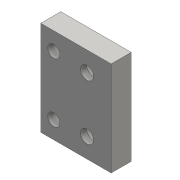
# Autodesk Inventor part: ROB-R-J-1
Saved by Autodesk Inventor 2016 (Build 200138000, 138)
## iProperties
Created: 2016-02-12
Part Number: ROB-R-J-1
Material: Generic
Document SubType Name: Modeling
Designer: admin
Density: 1 g/cm^3
Appearance: Default
Author: admin
Autodesk Inventor part; units mm, degrees
(part 1 of 3)
ref_plane "YZ Plane" through (0, 0, 0) normal (1, 0, 0) x (0, 1, 0)
ref_plane "XZ Plane" through (0, 0, 0) normal (0, 1, 0) x (-1, 0, 0)
ref_plane "XY Plane" through (0, 0, 0) normal (0, 0, 1) x (1, 0, 0)
sketch "Sketch1" plane through (0, 0, 0) normal (0, 1, 0) x (-1, 0, 0)
  spline S0 degree 3 poles (-66.561, 0) (-66.561, -4.1087) (-69.8644, -7.4121) (-73.9731, -7.4121) knots 0 0 0 0 1 1 1 1
  line L0 (-66.561, 0) -> (-66.561, -4.1087) construction
  line L1 (-66.561, -4.1087) -> (-69.8644, -7.4121) construction
  line L2 (-69.8644, -7.4121) -> (-73.9731, -7.4121) construction
  spline S1 degree 3 poles (-73.9731, -7.4121) (-78.0818, -7.4121) (-81.3852, -4.1087) (-81.3852, 0) knots 0 0 0 0 1 1 1 1
  line L3 (-73.9731, -7.4121) -> (-78.0818, -7.4121) construction
  line L4 (-78.0818, -7.4121) -> (-81.3852, -4.1087) construction
  line L5 (-81.3852, -4.1087) -> (-81.3852, 0) construction
  spline S2 degree 3 poles (-81.3852, 0) (-81.3852, 4.1087) (-78.0818, 7.4121) (-73.9731, 7.4121) knots 0 0 0 0 1 1 1 1
  line L6 (-81.3852, 0) -> (-81.3852, 4.1087) construction
  line L7 (-81.3852, 4.1087) -> (-78.0818, 7.4121) construction
  line L8 (-78.0818, 7.4121) -> (-73.9731, 7.4121) construction
  spline S3 degree 3 poles (-73.9731, 7.4121) (-69.8644, 7.4121) (-66.561, 4.1087) (-66.561, 0) knots 0 0 0 0 1 1 1 1
  line L9 (-73.9731, 7.4121) -> (-69.8644, 7.4121) construction
  line L10 (-69.8644, 7.4121) -> (-66.561, 4.1087) construction
  line L11 (-66.561, 4.1087) -> (-66.561, 0) construction
  spline S4 degree 3 poles (74.4391, 0) (74.4391, -4.1087) (71.1356, -7.4121) (67.027, -7.4121) knots 0 0 0 0 1 1 1 1
  line L12 (74.4391, 0) -> (74.4391, -4.1087) construction
  line L13 (74.4391, -4.1087) -> (71.1356, -7.4121) construction
  line L14 (71.1356, -7.4121) -> (67.027, -7.4121) construction
  spline S5 degree 3 poles (67.027, -7.4121) (62.9183, -7.4121) (59.6149, -4.1087) (59.6149, 0) knots 0 0 0 0 1 1 1 1
  line L15 (67.027, -7.4121) -> (62.9183, -7.4121) construction
  line L16 (62.9183, -7.4121) -> (59.6149, -4.1087) construction
  line L17 (59.6149, -4.1087) -> (59.6149, 0) construction
  spline S6 degree 3 poles (59.6149, 0) (59.6149, 4.1087) (62.9183, 7.4121) (67.027, 7.4121) knots 0 0 0 0 1 1 1 1
  line L18 (59.6149, 0) -> (59.6149, 4.1087) construction
  line L19 (59.6149, 4.1087) -> (62.9183, 7.4121) construction
  line L20 (62.9183, 7.4121) -> (67.027, 7.4121) construction
  spline S7 degree 3 poles (67.027, 7.4121) (71.1356, 7.4121) (74.4391, 4.1087) (74.4391, 0) knots 0 0 0 0 1 1 1 1
  line L21 (67.027, 7.4121) -> (71.1356, 7.4121) construction
  line L22 (71.1356, 7.4121) -> (74.4391, 4.1087) construction
  line L23 (74.4391, 4.1087) -> (74.4391, 0) construction
  spline S8 degree 3 poles (-60.9702, 4.9979) (-60.9702, 3.3462) (-62.3255, 1.9909) (-63.9772, 1.9909) knots 0 0 0 0 1 1 1 1
  line L24 (-60.9702, 4.9979) -> (-60.9702, 3.3462) construction
  line L25 (-60.9702, 3.3462) -> (-62.3255, 1.9909) construction
  line L26 (-62.3255, 1.9909) -> (-63.9772, 1.9909) construction
  spline S9 degree 3 poles (-63.9772, 1.9909) (-65.6289, 1.9909) (-66.9842, 3.3462) (-66.9842, 4.9979) knots 0 0 0 0 1 1 1 1
  line L27 (-63.9772, 1.9909) -> (-65.6289, 1.9909) construction
  line L28 (-65.6289, 1.9909) -> (-66.9842, 3.3462) construction
  line L29 (-66.9842, 3.3462) -> (-66.9842, 4.9979) construction
  spline S10 degree 3 poles (-66.9842, 4.9979) (-66.9842, 6.6497) (-65.6289, 8.005) (-63.9772, 8.005) knots 0 0 0 0 1 1 1 1
  line L30 (-66.9842, 4.9979) -> (-66.9842, 6.6497) construction
  line L31 (-66.9842, 6.6497) -> (-65.6289, 8.005) construction
  line L32 (-65.6289, 8.005) -> (-63.9772, 8.005) construction
  spline S11 degree 3 poles (-63.9772, 8.005) (-62.3255, 8.005) (-60.9702, 6.6497) (-60.9702, 4.9979) knots 0 0 0 0 1 1 1 1
  line L33 (-63.9772, 8.005) -> (-62.3255, 8.005) construction
  line L34 (-62.3255, 8.005) -> (-60.9702, 6.6497) construction
  line L35 (-60.9702, 6.6497) -> (-60.9702, 4.9979) construction
  spline S12 degree 3 poles (-50.9743, 4.9979) (-50.9743, 3.3462) (-52.3296, 1.9909) (-53.9813, 1.9909) knots 0 0 0 0 1 1 1 1
  line L36 (-50.9743, 4.9979) -> (-50.9743, 3.3462) construction
  line L37 (-50.9743, 3.3462) -> (-52.3296, 1.9909) construction
  line L38 (-52.3296, 1.9909) -> (-53.9813, 1.9909) construction
  spline S13 degree 3 poles (-53.9813, 1.9909) (-55.633, 1.9909) (-56.9883, 3.3462) (-56.9883, 4.9979) knots 0 0 0 0 1 1 1 1
  line L39 (-53.9813, 1.9909) -> (-55.633, 1.9909) construction
  line L40 (-55.633, 1.9909) -> (-56.9883, 3.3462) construction
  line L41 (-56.9883, 3.3462) -> (-56.9883, 4.9979) construction
  spline S14 degree 3 poles (-56.9883, 4.9979) (-56.9883, 6.6497) (-55.633, 8.005) (-53.9813, 8.005) knots 0 0 0 0 1 1 1 1
  line L42 (-56.9883, 4.9979) -> (-56.9883, 6.6497) construction
  line L43 (-56.9883, 6.6497) -> (-55.633, 8.005) construction
  line L44 (-55.633, 8.005) -> (-53.9813, 8.005) construction
  spline S15 degree 3 poles (-53.9813, 8.005) (-52.3296, 8.005) (-50.9743, 6.6497) (-50.9743, 4.9979) knots 0 0 0 0 1 1 1 1
  line L45 (-53.9813, 8.005) -> (-52.3296, 8.005) construction
  line L46 (-52.3296, 8.005) -> (-50.9743, 6.6497) construction
  line L47 (-50.9743, 6.6497) -> (-50.9743, 4.9979) construction
  spline S16 degree 3 poles (-50.9743, -4.998) (-50.9743, -6.6497) (-52.3296, -8.005) (-53.9813, -8.005) knots 0 0 0 0 1 1 1 1
  line L48 (-50.9743, -4.998) -> (-50.9743, -6.6497) construction
  line L49 (-50.9743, -6.6497) -> (-52.3296, -8.005) construction
  line L50 (-52.3296, -8.005) -> (-53.9813, -8.005) construction
  spline S17 degree 3 poles (-53.9813, -8.005) (-55.633, -8.005) (-56.9883, -6.6497) (-56.9883, -4.998) knots 0 0 0 0 1 1 1 1
  line L51 (-53.9813, -8.005) -> (-55.633, -8.005) construction
  line L52 (-55.633, -8.005) -> (-56.9883, -6.6497) construction
  line L53 (-56.9883, -6.6497) -> (-56.9883, -4.998) construction
  spline S18 degree 3 poles (-56.9883, -4.998) (-56.9883, -3.3462) (-55.633, -1.9909) (-53.9813, -1.9909) knots 0 0 0 0 1 1 1 1
  line L54 (-56.9883, -4.998) -> (-56.9883, -3.3462) construction
  line L55 (-56.9883, -3.3462) -> (-55.633, -1.9909) construction
  line L56 (-55.633, -1.9909) -> (-53.9813, -1.9909) construction
  spline S19 degree 3 poles (-53.9813, -1.9909) (-52.3296, -1.9909) (-50.9743, -3.3462) (-50.9743, -4.998) knots 0 0 0 0 1 1 1 1
  line L57 (-53.9813, -1.9909) -> (-52.3296, -1.9909) construction
  line L58 (-52.3296, -1.9909) -> (-50.9743, -3.3462) construction
  line L59 (-50.9743, -3.3462) -> (-50.9743, -4.998) construction
  spline S20 degree 3 poles (-60.9702, -4.998) (-60.9702, -6.6497) (-62.3255, -8.005) (-63.9772, -8.005) knots 0 0 0 0 1 1 1 1
  line L60 (-60.9702, -4.998) -> (-60.9702, -6.6497) construction
  line L61 (-60.9702, -6.6497) -> (-62.3255, -8.005) construction
  line L62 (-62.3255, -8.005) -> (-63.9772, -8.005) construction
  spline S21 degree 3 poles (-63.9772, -8.005) (-65.6289, -8.005) (-66.9842, -6.6497) (-66.9842, -4.998) knots 0 0 0 0 1 1 1 1
  line L63 (-63.9772, -8.005) -> (-65.6289, -8.005) construction
  line L64 (-65.6289, -8.005) -> (-66.9842, -6.6497) construction
  line L65 (-66.9842, -6.6497) -> (-66.9842, -4.998) construction
  spline S22 degree 3 poles (-66.9842, -4.998) (-66.9842, -3.3462) (-65.6289, -1.9909) (-63.9772, -1.9909) knots 0 0 0 0 1 1 1 1
  line L66 (-66.9842, -4.998) -> (-66.9842, -3.3462) construction
  line L67 (-66.9842, -3.3462) -> (-65.6289, -1.9909) construction
  line L68 (-65.6289, -1.9909) -> (-63.9772, -1.9909) construction
  spline S23 degree 3 poles (-63.9772, -1.9909) (-62.3255, -1.9909) (-60.9702, -3.3462) (-60.9702, -4.998) knots 0 0 0 0 1 1 1 1
  line L69 (-63.9772, -1.9909) -> (-62.3255, -1.9909) construction
  line L70 (-62.3255, -1.9909) -> (-60.9702, -3.3462) construction
  line L71 (-60.9702, -3.3462) -> (-60.9702, -4.998) construction
  spline S24 degree 3 poles (-38.9875, 40.025) (-38.9875, 38.3732) (-40.3428, 37.0179) (-41.9945, 37.0179) knots 0 0 0 0 1 1 1 1
  line L72 (-38.9875, 40.025) -> (-38.9875, 38.3732) construction
  line L73 (-38.9875, 38.3732) -> (-40.3428, 37.0179) construction
  line L74 (-40.3428, 37.0179) -> (-41.9945, 37.0179) construction
  spline S25 degree 3 poles (-41.9945, 37.0179) (-43.6462, 37.0179) (-45.0015, 38.3732) (-45.0015, 40.025) knots 0 0 0 0 1 1 1 1
  line L75 (-41.9945, 37.0179) -> (-43.6462, 37.0179) construction
  line L76 (-43.6462, 37.0179) -> (-45.0015, 38.3732) construction
  line L77 (-45.0015, 38.3732) -> (-45.0015, 40.025) construction
  spline S26 degree 3 poles (-45.0015, 40.025) (-45.0015, 41.6767) (-43.6462, 43.032) (-41.9945, 43.032) knots 0 0 0 0 1 1 1 1
  line L78 (-45.0015, 40.025) -> (-45.0015, 41.6767) construction
  line L79 (-45.0015, 41.6767) -> (-43.6462, 43.032) construction
  line L80 (-43.6462, 43.032) -> (-41.9945, 43.032) construction
  spline S27 degree 3 poles (-41.9945, 43.032) (-40.3428, 43.032) (-38.9875, 41.6767) (-38.9875, 40.025) knots 0 0 0 0 1 1 1 1
  line L81 (-41.9945, 43.032) -> (-40.3428, 43.032) construction
  line L82 (-40.3428, 43.032) -> (-38.9875, 41.6767) construction
  line L83 (-38.9875, 41.6767) -> (-38.9875, 40.025) construction
  spline S28 degree 3 poles (-28.9916, 40.025) (-28.9916, 38.3732) (-30.3469, 37.0179) (-31.9986, 37.0179) knots 0 0 0 0 1 1 1 1
  line L84 (-28.9916, 40.025) -> (-28.9916, 38.3732) construction
  line L85 (-28.9916, 38.3732) -> (-30.3469, 37.0179) construction
  line L86 (-30.3469, 37.0179) -> (-31.9986, 37.0179) construction
  spline S29 degree 3 poles (-31.9986, 37.0179) (-33.6503, 37.0179) (-35.0056, 38.3732) (-35.0056, 40.025) knots 0 0 0 0 1 1 1 1
  line L87 (-31.9986, 37.0179) -> (-33.6503, 37.0179) construction
  line L88 (-33.6503, 37.0179) -> (-35.0056, 38.3732) construction
  line L89 (-35.0056, 38.3732) -> (-35.0056, 40.025) construction
  spline S30 degree 3 poles (-35.0056, 40.025) (-35.0056, 41.6767) (-33.6503, 43.032) (-31.9986, 43.032) knots 0 0 0 0 1 1 1 1
  line L90 (-35.0056, 40.025) -> (-35.0056, 41.6767) construction
  line L91 (-35.0056, 41.6767) -> (-33.6503, 43.032) construction
  line L92 (-33.6503, 43.032) -> (-31.9986, 43.032) construction
  spline S31 degree 3 poles (-31.9986, 43.032) (-30.3469, 43.032) (-28.9916, 41.6767) (-28.9916, 40.025) knots 0 0 0 0 1 1 1 1
  line L93 (-31.9986, 43.032) -> (-30.3469, 43.032) construction
  line L94 (-30.3469, 43.032) -> (-28.9916, 41.6767) construction
  line L95 (-28.9916, 41.6767) -> (-28.9916, 40.025) construction
  spline S32 degree 3 poles (-28.9916, 30.0291) (-28.9916, 28.3773) (-30.3469, 27.022) (-31.9986, 27.022) knots 0 0 0 0 1 1 1 1
  line L96 (-28.9916, 30.0291) -> (-28.9916, 28.3773) construction
  line L97 (-28.9916, 28.3773) -> (-30.3469, 27.022) construction
  line L98 (-30.3469, 27.022) -> (-31.9986, 27.022) construction
  spline S33 degree 3 poles (-31.9986, 27.022) (-33.6503, 27.022) (-35.0056, 28.3773) (-35.0056, 30.0291) knots 0 0 0 0 1 1 1 1
  line L99 (-31.9986, 27.022) -> (-33.6503, 27.022) construction
  line L100 (-33.6503, 27.022) -> (-35.0056, 28.3773) construction
  line L101 (-35.0056, 28.3773) -> (-35.0056, 30.0291) construction
  spline S34 degree 3 poles (-35.0056, 30.0291) (-35.0056, 31.6808) (-33.6503, 33.0361) (-31.9986, 33.0361) knots 0 0 0 0 1 1 1 1
  line L102 (-35.0056, 30.0291) -> (-35.0056, 31.6808) construction
  line L103 (-35.0056, 31.6808) -> (-33.6503, 33.0361) construction
  line L104 (-33.6503, 33.0361) -> (-31.9986, 33.0361) construction
  spline S35 degree 3 poles (-31.9986, 33.0361) (-30.3469, 33.0361) (-28.9916, 31.6808) (-28.9916, 30.0291) knots 0 0 0 0 1 1 1 1
  line L105 (-31.9986, 33.0361) -> (-30.3469, 33.0361) construction
  line L106 (-30.3469, 33.0361) -> (-28.9916, 31.6808) construction
  line L107 (-28.9916, 31.6808) -> (-28.9916, 30.0291) construction
  spline S36 degree 3 poles (-38.9875, 30.0291) (-38.9875, 28.3773) (-40.3428, 27.022) (-41.9945, 27.022) knots 0 0 0 0 1 1 1 1
  line L108 (-38.9875, 30.0291) -> (-38.9875, 28.3773) construction
  line L109 (-38.9875, 28.3773) -> (-40.3428, 27.022) construction
  line L110 (-40.3428, 27.022) -> (-41.9945, 27.022) construction
  spline S37 degree 3 poles (-41.9945, 27.022) (-43.6462, 27.022) (-45.0015, 28.3773) (-45.0015, 30.0291) knots 0 0 0 0 1 1 1 1
  line L111 (-41.9945, 27.022) -> (-43.6462, 27.022) construction
  line L112 (-43.6462, 27.022) -> (-45.0015, 28.3773) construction
  line L113 (-45.0015, 28.3773) -> (-45.0015, 30.0291) construction
  spline S38 degree 3 poles (-45.0015, 30.0291) (-45.0015, 31.6808) (-43.6462, 33.0361) (-41.9945, 33.0361) knots 0 0 0 0 1 1 1 1
  line L114 (-45.0015, 30.0291) -> (-45.0015, 31.6808) construction
  line L115 (-45.0015, 31.6808) -> (-43.6462, 33.0361) construction
  line L116 (-43.6462, 33.0361) -> (-41.9945, 33.0361) construction
  spline S39 degree 3 poles (-41.9945, 33.0361) (-40.3428, 33.0361) (-38.9875, 31.6808) (-38.9875, 30.0291) knots 0 0 0 0 1 1 1 1
  line L117 (-41.9945, 33.0361) -> (-40.3428, 33.0361) construction
  line L118 (-40.3428, 33.0361) -> (-38.9875, 31.6808) construction
  line L119 (-38.9875, 31.6808) -> (-38.9875, 30.0291) construction
  spline S40 degree 3 poles (44.0281, 30.0291) (44.0281, 28.3773) (42.6728, 27.022) (41.0211, 27.022) knots 0 0 0 0 1 1 1 1
  line L120 (44.0281, 30.0291) -> (44.0281, 28.3773) construction
  line L121 (44.0281, 28.3773) -> (42.6728, 27.022) construction
  line L122 (42.6728, 27.022) -> (41.0211, 27.022) construction
  spline S41 degree 3 poles (41.0211, 27.022) (39.3694, 27.022) (38.0141, 28.3773) (38.0141, 30.0291) knots 0 0 0 0 1 1 1 1
  line L123 (41.0211, 27.022) -> (39.3694, 27.022) construction
  line L124 (39.3694, 27.022) -> (38.0141, 28.3773) construction
  line L125 (38.0141, 28.3773) -> (38.0141, 30.0291) construction
  spline S42 degree 3 poles (38.0141, 30.0291) (38.0141, 31.6808) (39.3694, 33.0361) (41.0211, 33.0361) knots 0 0 0 0 1 1 1 1
  line L126 (38.0141, 30.0291) -> (38.0141, 31.6808) construction
  line L127 (38.0141, 31.6808) -> (39.3694, 33.0361) construction
  line L128 (39.3694, 33.0361) -> (41.0211, 33.0361) construction
  spline S43 degree 3 poles (41.0211, 33.0361) (42.6728, 33.0361) (44.0281, 31.6808) (44.0281, 30.0291) knots 0 0 0 0 1 1 1 1
  line L129 (41.0211, 33.0361) -> (42.6728, 33.0361) construction
  line L130 (42.6728, 33.0361) -> (44.0281, 31.6808) construction
  line L131 (44.0281, 31.6808) -> (44.0281, 30.0291) construction
  spline S44 degree 3 poles (34.0322, 30.0291) (34.0322, 28.3773) (32.6769, 27.022) (31.0252, 27.022) knots 0 0 0 0 1 1 1 1
  line L132 (34.0322, 30.0291) -> (34.0322, 28.3773) construction
  line L133 (34.0322, 28.3773) -> (32.6769, 27.022) construction
  line L134 (32.6769, 27.022) -> (31.0252, 27.022) construction
  spline S45 degree 3 poles (31.0252, 27.022) (29.3735, 27.022) (28.0182, 28.3773) (28.0182, 30.0291) knots 0 0 0 0 1 1 1 1
  line L135 (31.0252, 27.022) -> (29.3735, 27.022) construction
  line L136 (29.3735, 27.022) -> (28.0182, 28.3773) construction
  line L137 (28.0182, 28.3773) -> (28.0182, 30.0291) construction
  spline S46 degree 3 poles (28.0182, 30.0291) (28.0182, 31.6808) (29.3735, 33.0361) (31.0252, 33.0361) knots 0 0 0 0 1 1 1 1
  line L138 (28.0182, 30.0291) -> (28.0182, 31.6808) construction
  line L139 (28.0182, 31.6808) -> (29.3735, 33.0361) construction
  line L140 (29.3735, 33.0361) -> (31.0252, 33.0361) construction
  spline S47 degree 3 poles (31.0252, 33.0361) (32.6769, 33.0361) (34.0322, 31.6808) (34.0322, 30.0291) knots 0 0 0 0 1 1 1 1
  line L141 (31.0252, 33.0361) -> (32.6769, 33.0361) construction
  line L142 (32.6769, 33.0361) -> (34.0322, 31.6808) construction
  line L143 (34.0322, 31.6808) -> (34.0322, 30.0291) construction
  spline S48 degree 3 poles (34.0322, 40.025) (34.0322, 38.3732) (32.6769, 37.0179) (31.0252, 37.0179) knots 0 0 0 0 1 1 1 1
  line L144 (34.0322, 40.025) -> (34.0322, 38.3732) construction
  line L145 (34.0322, 38.3732) -> (32.6769, 37.0179) construction
  line L146 (32.6769, 37.0179) -> (31.0252, 37.0179) construction
  spline S49 degree 3 poles (31.0252, 37.0179) (29.3735, 37.0179) (28.0182, 38.3732) (28.0182, 40.025) knots 0 0 0 0 1 1 1 1
  line L147 (31.0252, 37.0179) -> (29.3735, 37.0179) construction
  line L148 (29.3735, 37.0179) -> (28.0182, 38.3732) construction
  line L149 (28.0182, 38.3732) -> (28.0182, 40.025) construction
  spline S50 degree 3 poles (28.0182, 40.025) (28.0182, 41.6767) (29.3735, 43.032) (31.0252, 43.032) knots 0 0 0 0 1 1 1 1
  line L150 (28.0182, 40.025) -> (28.0182, 41.6767) construction
  line L151 (28.0182, 41.6767) -> (29.3735, 43.032) construction
  line L152 (29.3735, 43.032) -> (31.0252, 43.032) construction
  spline S51 degree 3 poles (31.0252, 43.032) (32.6769, 43.032) (34.0322, 41.6767) (34.0322, 40.025) knots 0 0 0 0 1 1 1 1
  line L153 (31.0252, 43.032) -> (32.6769, 43.032) construction
  line L154 (32.6769, 43.032) -> (34.0322, 41.6767) construction
  line L155 (34.0322, 41.6767) -> (34.0322, 40.025) construction
  spline S52 degree 3 poles (44.0281, 40.025) (44.0281, 38.3732) (42.6728, 37.0179) (41.0211, 37.0179) knots 0 0 0 0 1 1 1 1
  line L156 (44.0281, 40.025) -> (44.0281, 38.3732) construction
  line L157 (44.0281, 38.3732) -> (42.6728, 37.0179) construction
  line L158 (42.6728, 37.0179) -> (41.0211, 37.0179) construction
  spline S53 degree 3 poles (41.0211, 37.0179) (39.3694, 37.0179) (38.0141, 38.3732) (38.0141, 40.025) knots 0 0 0 0 1 1 1 1
  line L159 (41.0211, 37.0179) -> (39.3694, 37.0179) construction
  line L160 (39.3694, 37.0179) -> (38.0141, 38.3732) construction
  line L161 (38.0141, 38.3732) -> (38.0141, 40.025) construction
  spline S54 degree 3 poles (38.0141, 40.025) (38.0141, 41.6767) (39.3694, 43.032) (41.0211, 43.032) knots 0 0 0 0 1 1 1 1
  line L162 (38.0141, 40.025) -> (38.0141, 41.6767) construction
  line L163 (38.0141, 41.6767) -> (39.3694, 43.032) construction
  line L164 (39.3694, 43.032) -> (41.0211, 43.032) construction
  spline S55 degree 3 poles (41.0211, 43.032) (42.6728, 43.032) (44.0281, 41.6767) (44.0281, 40.025) knots 0 0 0 0 1 1 1 1
  line L165 (41.0211, 43.032) -> (42.6728, 43.032) construction
  line L166 (42.6728, 43.032) -> (44.0281, 41.6767) construction
  line L167 (44.0281, 41.6767) -> (44.0281, 40.025) construction
  spline S56 degree 3 poles (44.0281, -39.9836) (44.0281, -41.6353) (42.6728, -42.9906) (41.0211, -42.9906) knots 0 0 0 0 1 1 1 1
  line L168 (44.0281, -39.9836) -> (44.0281, -41.6353) construction
  line L169 (44.0281, -41.6353) -> (42.6728, -42.9906) construction
  line L170 (42.6728, -42.9906) -> (41.0211, -42.9906) construction
  spline S57 degree 3 poles (41.0211, -42.9906) (39.3694, -42.9906) (38.0141, -41.6353) (38.0141, -39.9836) knots 0 0 0 0 1 1 1 1
  line L171 (41.0211, -42.9906) -> (39.3694, -42.9906) construction
  line L172 (39.3694, -42.9906) -> (38.0141, -41.6353) construction
  line L173 (38.0141, -41.6353) -> (38.0141, -39.9836) construction
  spline S58 degree 3 poles (38.0141, -39.9836) (38.0141, -38.3319) (39.3694, -36.9766) (41.0211, -36.9766) knots 0 0 0 0 1 1 1 1
  line L174 (38.0141, -39.9836) -> (38.0141, -38.3319) construction
  line L175 (38.0141, -38.3319) -> (39.3694, -36.9766) construction
  line L176 (39.3694, -36.9766) -> (41.0211, -36.9766) construction
  spline S59 degree 3 poles (41.0211, -36.9766) (42.6728, -36.9766) (44.0281, -38.3319) (44.0281, -39.9836) knots 0 0 0 0 1 1 1 1
  line L177 (41.0211, -36.9766) -> (42.6728, -36.9766) construction
  line L178 (42.6728, -36.9766) -> (44.0281, -38.3319) construction
  line L179 (44.0281, -38.3319) -> (44.0281, -39.9836) construction
  spline S60 degree 3 poles (34.0322, -39.9836) (34.0322, -41.6353) (32.6769, -42.9906) (31.0252, -42.9906) knots 0 0 0 0 1 1 1 1
  line L180 (34.0322, -39.9836) -> (34.0322, -41.6353) construction
  line L181 (34.0322, -41.6353) -> (32.6769, -42.9906) construction
  line L182 (32.6769, -42.9906) -> (31.0252, -42.9906) construction
  spline S61 degree 3 poles (31.0252, -42.9906) (29.3735, -42.9906) (28.0182, -41.6353) (28.0182, -39.9836) knots 0 0 0 0 1 1 1 1
  line L183 (31.0252, -42.9906) -> (29.3735, -42.9906) construction
  line L184 (29.3735, -42.9906) -> (28.0182, -41.6353) construction
  line L185 (28.0182, -41.6353) -> (28.0182, -39.9836) construction
  spline S62 degree 3 poles (28.0182, -39.9836) (28.0182, -38.3319) (29.3735, -36.9766) (31.0252, -36.9766) knots 0 0 0 0 1 1 1 1
  line L186 (28.0182, -39.9836) -> (28.0182, -38.3319) construction
  line L187 (28.0182, -38.3319) -> (29.3735, -36.9766) construction
  line L188 (29.3735, -36.9766) -> (31.0252, -36.9766) construction
  spline S63 degree 3 poles (31.0252, -36.9766) (32.6769, -36.9766) (34.0322, -38.3319) (34.0322, -39.9836) knots 0 0 0 0 1 1 1 1
  line L189 (31.0252, -36.9766) -> (32.6769, -36.9766) construction
  line L190 (32.6769, -36.9766) -> (34.0322, -38.3319) construction
  line L191 (34.0322, -38.3319) -> (34.0322, -39.9836) construction
  spline S64 degree 3 poles (34.0322, -29.9877) (34.0322, -31.6394) (32.6769, -32.9947) (31.0252, -32.9947) knots 0 0 0 0 1 1 1 1
  line L192 (34.0322, -29.9877) -> (34.0322, -31.6394) construction
  line L193 (34.0322, -31.6394) -> (32.6769, -32.9947) construction
  line L194 (32.6769, -32.9947) -> (31.0252, -32.9947) construction
  spline S65 degree 3 poles (31.0252, -32.9947) (29.3735, -32.9947) (28.0182, -31.6394) (28.0182, -29.9877) knots 0 0 0 0 1 1 1 1
  line L195 (31.0252, -32.9947) -> (29.3735, -32.9947) construction
  line L196 (29.3735, -32.9947) -> (28.0182, -31.6394) construction
  line L197 (28.0182, -31.6394) -> (28.0182, -29.9877) construction
  spline S66 degree 3 poles (28.0182, -29.9877) (28.0182, -28.336) (29.3735, -26.9807) (31.0252, -26.9807) knots 0 0 0 0 1 1 1 1
  line L198 (28.0182, -29.9877) -> (28.0182, -28.336) construction
  line L199 (28.0182, -28.336) -> (29.3735, -26.9807) construction
  line L200 (29.3735, -26.9807) -> (31.0252, -26.9807) construction
  spline S67 degree 3 poles (31.0252, -26.9807) (32.6769, -26.9807) (34.0322, -28.336) (34.0322, -29.9877) knots 0 0 0 0 1 1 1 1
  line L201 (31.0252, -26.9807) -> (32.6769, -26.9807) construction
  line L202 (32.6769, -26.9807) -> (34.0322, -28.336) construction
  line L203 (34.0322, -28.336) -> (34.0322, -29.9877) construction
  spline S68 degree 3 poles (44.0281, -29.9877) (44.0281, -31.6394) (42.6728, -32.9947) (41.0211, -32.9947) knots 0 0 0 0 1 1 1 1
  line L204 (44.0281, -29.9877) -> (44.0281, -31.6394) construction
  line L205 (44.0281, -31.6394) -> (42.6728, -32.9947) construction
  line L206 (42.6728, -32.9947) -> (41.0211, -32.9947) construction
  spline S69 degree 3 poles (41.0211, -32.9947) (39.3694, -32.9947) (38.0141, -31.6394) (38.0141, -29.9877) knots 0 0 0 0 1 1 1 1
  line L207 (41.0211, -32.9947) -> (39.3694, -32.9947) construction
  line L208 (39.3694, -32.9947) -> (38.0141, -31.6394) construction
  line L209 (38.0141, -31.6394) -> (38.0141, -29.9877) construction
  spline S70 degree 3 poles (38.0141, -29.9877) (38.0141, -28.336) (39.3694, -26.9807) (41.0211, -26.9807) knots 0 0 0 0 1 1 1 1
  line L210 (38.0141, -29.9877) -> (38.0141, -28.336) construction
  line L211 (38.0141, -28.336) -> (39.3694, -26.9807) construction
  line L212 (39.3694, -26.9807) -> (41.0211, -26.9807) construction
  spline S71 degree 3 poles (41.0211, -26.9807) (42.6728, -26.9807) (44.0281, -28.336) (44.0281, -29.9877) knots 0 0 0 0 1 1 1 1
  line L213 (41.0211, -26.9807) -> (42.6728, -26.9807) construction
  line L214 (42.6728, -26.9807) -> (44.0281, -28.336) construction
  line L215 (44.0281, -28.336) -> (44.0281, -29.9877) construction
  spline S72 degree 3 poles (-38.9875, -29.9877) (-38.9875, -31.6394) (-40.3428, -32.9947) (-41.9945, -32.9947) knots 0 0 0 0 1 1 1 1
  line L216 (-38.9875, -29.9877) -> (-38.9875, -31.6394) construction
  line L217 (-38.9875, -31.6394) -> (-40.3428, -32.9947) construction
  line L218 (-40.3428, -32.9947) -> (-41.9945, -32.9947) construction
  spline S73 degree 3 poles (-41.9945, -32.9947) (-43.6462, -32.9947) (-45.0015, -31.6394) (-45.0015, -29.9877) knots 0 0 0 0 1 1 1 1
  line L219 (-41.9945, -32.9947) -> (-43.6462, -32.9947) construction
  line L220 (-43.6462, -32.9947) -> (-45.0015, -31.6394) construction
  line L221 (-45.0015, -31.6394) -> (-45.0015, -29.9877) construction
  spline S74 degree 3 poles (-45.0015, -29.9877) (-45.0015, -28.336) (-43.6462, -26.9807) (-41.9945, -26.9807) knots 0 0 0 0 1 1 1 1
  line L222 (-45.0015, -29.9877) -> (-45.0015, -28.336) construction
  line L223 (-45.0015, -28.336) -> (-43.6462, -26.9807) construction
  line L224 (-43.6462, -26.9807) -> (-41.9945, -26.9807) construction
  spline S75 degree 3 poles (-41.9945, -26.9807) (-40.3428, -26.9807) (-38.9875, -28.336) (-38.9875, -29.9877) knots 0 0 0 0 1 1 1 1
  line L225 (-41.9945, -26.9807) -> (-40.3428, -26.9807) construction
  line L226 (-40.3428, -26.9807) -> (-38.9875, -28.336) construction
  line L227 (-38.9875, -28.336) -> (-38.9875, -29.9877) construction
  spline S76 degree 3 poles (-28.9916, -29.9877) (-28.9916, -31.6394) (-30.3469, -32.9947) (-31.9986, -32.9947) knots 0 0 0 0 1 1 1 1
  line L228 (-28.9916, -29.9877) -> (-28.9916, -31.6394) construction
  line L229 (-28.9916, -31.6394) -> (-30.3469, -32.9947) construction
  line L230 (-30.3469, -32.9947) -> (-31.9986, -32.9947) construction
  spline S77 degree 3 poles (-31.9986, -32.9947) (-33.6503, -32.9947) (-35.0056, -31.6394) (-35.0056, -29.9877) knots 0 0 0 0 1 1 1 1
  line L231 (-31.9986, -32.9947) -> (-33.6503, -32.9947) construction
  line L232 (-33.6503, -32.9947) -> (-35.0056, -31.6394) construction
  line L233 (-35.0056, -31.6394) -> (-35.0056, -29.9877) construction
  spline S78 degree 3 poles (-35.0056, -29.9877) (-35.0056, -28.336) (-33.6503, -26.9807) (-31.9986, -26.9807) knots 0 0 0 0 1 1 1 1
  line L234 (-35.0056, -29.9877) -> (-35.0056, -28.336) construction
  line L235 (-35.0056, -28.336) -> (-33.6503, -26.9807) construction
  line L236 (-33.6503, -26.9807) -> (-31.9986, -26.9807) construction
  spline S79 degree 3 poles (-31.9986, -26.9807) (-30.3469, -26.9807) (-28.9916, -28.336) (-28.9916, -29.9877) knots 0 0 0 0 1 1 1 1
  line L237 (-31.9986, -26.9807) -> (-30.3469, -26.9807) construction
  line L238 (-30.3469, -26.9807) -> (-28.9916, -28.336) construction
  line L239 (-28.9916, -28.336) -> (-28.9916, -29.9877) construction
  spline S80 degree 3 poles (-28.9916, -39.9836) (-28.9916, -41.6353) (-30.3469, -42.9906) (-31.9986, -42.9906) knots 0 0 0 0 1 1 1 1
  line L240 (-28.9916, -39.9836) -> (-28.9916, -41.6353) construction
  line L241 (-28.9916, -41.6353) -> (-30.3469, -42.9906) construction
  line L242 (-30.3469, -42.9906) -> (-31.9986, -42.9906) construction
  spline S81 degree 3 poles (-31.9986, -42.9906) (-33.6503, -42.9906) (-35.0056, -41.6353) (-35.0056, -39.9836) knots 0 0 0 0 1 1 1 1
  line L243 (-31.9986, -42.9906) -> (-33.6503, -42.9906) construction
  line L244 (-33.6503, -42.9906) -> (-35.0056, -41.6353) construction
  line L245 (-35.0056, -41.6353) -> (-35.0056, -39.9836) construction
  spline S82 degree 3 poles (-35.0056, -39.9836) (-35.0056, -38.3319) (-33.6503, -36.9766) (-31.9986, -36.9766) knots 0 0 0 0 1 1 1 1
  line L246 (-35.0056, -39.9836) -> (-35.0056, -38.3319) construction
  line L247 (-35.0056, -38.3319) -> (-33.6503, -36.9766) construction
  line L248 (-33.6503, -36.9766) -> (-31.9986, -36.9766) construction
  spline S83 degree 3 poles (-31.9986, -36.9766) (-30.3469, -36.9766) (-28.9916, -38.3319) (-28.9916, -39.9836) knots 0 0 0 0 1 1 1 1
  line L249 (-31.9986, -36.9766) -> (-30.3469, -36.9766) construction
  line L250 (-30.3469, -36.9766) -> (-28.9916, -38.3319) construction
  line L251 (-28.9916, -38.3319) -> (-28.9916, -39.9836) construction
  spline S84 degree 3 poles (-38.9875, -39.9836) (-38.9875, -41.6353) (-40.3428, -42.9906) (-41.9945, -42.9906) knots 0 0 0 0 1 1 1 1
  line L252 (-38.9875, -39.9836) -> (-38.9875, -41.6353) construction
  line L253 (-38.9875, -41.6353) -> (-40.3428, -42.9906) construction
  line L254 (-40.3428, -42.9906) -> (-41.9945, -42.9906) construction
  spline S85 degree 3 poles (-41.9945, -42.9906) (-43.6462, -42.9906) (-45.0015, -41.6353) (-45.0015, -39.9836) knots 0 0 0 0 1 1 1 1
  line L255 (-41.9945, -42.9906) -> (-43.6462, -42.9906) construction
  line L256 (-43.6462, -42.9906) -> (-45.0015, -41.6353) construction
  line L257 (-45.0015, -41.6353) -> (-45.0015, -39.9836) construction
  spline S86 degree 3 poles (-45.0015, -39.9836) (-45.0015, -38.3319) (-43.6462, -36.9766) (-41.9945, -36.9766) knots 0 0 0 0 1 1 1 1
  line L258 (-45.0015, -39.9836) -> (-45.0015, -38.3319) construction
  line L259 (-45.0015, -38.3319) -> (-43.6462, -36.9766) construction
  line L260 (-43.6462, -36.9766) -> (-41.9945, -36.9766) construction
  spline S87 degree 3 poles (-41.9945, -36.9766) (-40.3428, -36.9766) (-38.9875, -38.3319) (-38.9875, -39.9836) knots 0 0 0 0 1 1 1 1
  line L261 (-41.9945, -36.9766) -> (-40.3428, -36.9766) construction
  line L262 (-40.3428, -36.9766) -> (-38.9875, -38.3319) construction
  line L263 (-38.9875, -38.3319) -> (-38.9875, -39.9836) construction
  line L264 (1.7158, 55.3993) -> (1.7158, 57.2207)
  line L265 (1.7158, 57.2207) -> (1.7158, 58.1113)
  line L266 (1.7158, 58.1113) -> (0.9107, 58.1113)
  line L267 (0.9107, 58.1113) -> (0.6997, 58.1113)
  line L268 (0.6997, 58.1113) -> (-0.8679, 58.1113)
  line L269 (-0.8679, 58.1113) -> (-1.6731, 58.1113)
  line L270 (-1.6731, 58.1113) -> (-1.6731, 55.3993)
  line L271 (-1.6731, 55.3993) -> (-0.8679, 55.3993)
  line L272 (-0.8679, 55.3993) -> (0.9107, 55.3993)
  line L273 (0.9107, 55.3993) -> (1.7158, 55.3993)
  line L274 (0.6997, 58.1113) -> (1.7158, 57.2207)
  line L275 (0.9107, 55.3993) -> (0.9107, 54.4259)
  line L276 (0.9107, 58.1113) -> (0.9107, 59.2116)
  line L277 (-0.8679, 58.1113) -> (-0.8679, 59.2116)
  line L278 (-0.8679, 55.3993) -> (-0.8679, 54.4259)
  line L279 (1.7158, -58.1968) -> (1.7158, -56.3755)
  line L280 (1.7158, -56.3755) -> (1.7158, -55.4848)
  line L281 (1.7158, -55.4848) -> (0.9107, -55.4848)
  line L282 (0.9107, -55.4848) -> (0.6997, -55.4848)
  line L283 (0.6997, -55.4848) -> (-0.8679, -55.4848)
  line L284 (-0.8679, -55.4848) -> (-1.6731, -55.4848)
  line L285 (-1.6731, -55.4848) -> (-1.6731, -58.1968)
  line L286 (-1.6731, -58.1968) -> (-0.8679, -58.1968)
  line L287 (-0.8679, -58.1968) -> (0.9107, -58.1968)
  line L288 (0.9107, -58.1968) -> (1.7158, -58.1968)
  line L289 (0.6997, -55.4848) -> (1.7158, -56.3755)
  line L290 (0.9107, -58.1968) -> (0.9107, -59.1702)
  line L291 (0.9107, -55.4848) -> (0.9107, -54.3846)
  line L292 (-0.8679, -55.4848) -> (-0.8679, -54.3846)
  line L293 (-0.8679, -58.1968) -> (-0.8679, -59.1702)
  line L294 (-43.5621, -3.3035) -> (-44.7906, -3.3035)
  line L295 (-44.7906, -3.3035) -> (-44.7906, -2.7106)
  line L296 (-44.7906, -2.7106) -> (-44.5783, -2.4997)
  line L297 (-44.5783, -2.4997) -> (-44.1977, -2.4997)
  line L298 (-44.1977, -2.4997) -> (-43.9854, -2.7106)
  line L299 (-43.9854, -2.7106) -> (-43.9854, -3.3035)
  line L300 (-44.7906, -1.398) -> (-44.7906, -1.8213)
  line L301 (-44.7906, -1.8213) -> (-44.5783, -1.9909)
  line L302 (-44.5783, -1.9909) -> (-43.7731, -1.9909)
  line L303 (-43.7731, -1.9909) -> (-43.5621, -1.8213)
  line L304 (-43.5621, -1.8213) -> (-43.5621, -1.398)
  line L305 (-43.5621, -1.398) -> (-43.7731, -1.1857)
  line L306 (-43.7731, -1.1857) -> (-44.5783, -1.1857)
  line L307 (-44.5783, -1.1857) -> (-44.7906, -1.398)
  line L308 (-44.7906, -0.6783) -> (-43.5621, -0.6783)
  line L309 (-43.5621, -0.6783) -> (-43.9854, -0.2964)
  line L310 (-43.9854, -0.2964) -> (-43.5621, 0.1268)
  line L311 (-43.5621, 0.1268) -> (-44.7906, 0.1268)
  line L312 (-44.7906, 1.4394) -> (-44.7906, 0.5929)
  line L313 (-44.7906, 0.5929) -> (-43.5621, 0.5929)
  line L314 (-43.5621, 0.5929) -> (-43.5621, 1.4394)
  line L315 (-44.1977, 0.5929) -> (-44.1977, 1.0161)
  line L316 (-43.5621, 1.9054) -> (-44.7906, 1.9054)
  line L317 (-44.7906, 1.9054) -> (-44.7906, 2.541)
  line L318 (-44.7906, 2.541) -> (-44.5783, 2.7533)
  line L319 (-44.5783, 2.7533) -> (-44.1977, 2.7533)
  line L320 (-44.1977, 2.7533) -> (-43.9854, 2.541)
  line L321 (-43.9854, 2.541) -> (-43.9854, 1.9054)
  line L322 (-43.9854, 2.3287) -> (-43.5621, 2.7533)
  line L323 (-44.7906, 5.1675) -> (-44.7906, 4.7429)
  line L324 (-44.7906, 4.7429) -> (-44.5783, 4.5319)
  line L325 (-44.5783, 4.5319) -> (-43.7731, 4.5319)
  line L326 (-43.7731, 4.5319) -> (-43.5621, 4.7429)
  line L327 (-43.5621, 4.7429) -> (-43.5621, 5.1675)
  line L328 (-43.5621, 5.1675) -> (-43.7731, 5.3357)
  line L329 (-43.7731, 5.3357) -> (-44.5783, 5.3357)
  line L330 (-44.5783, 5.3357) -> (-44.7906, 5.1675)
  line L331 (-43.5621, 5.8445) -> (-44.7906, 5.8445)
  line L332 (-44.7906, 5.8445) -> (-43.5621, 6.6497)
  line L333 (-43.5621, 6.6497) -> (-44.7906, 6.6497)
  line L334 (-37.5894, 10.3337) -> (-37.8017, 10.1227)
  line L335 (-37.8017, 10.1227) -> (-37.8017, 9.6995)
  line L336 (-37.8017, 9.6995) -> (-37.5894, 9.5299)
  line L337 (-37.5894, 9.5299) -> (-37.3785, 9.5299)
  line L338 (-37.3785, 9.5299) -> (-37.1661, 9.6995)
  line L339 (-37.1661, 9.6995) -> (-37.1661, 10.1227)
  line L340 (-37.1661, 10.1227) -> (-36.9965, 10.3337)
  line L341 (-36.9965, 10.3337) -> (-36.7856, 10.3337)
  line L342 (-36.7856, 10.3337) -> (-36.5733, 10.1227)
  line L343 (-36.5733, 10.1227) -> (-36.5733, 9.6995)
  line L344 (-36.5733, 9.6995) -> (-36.7856, 9.5299)
  line L345 (-36.5733, 11.2244) -> (-37.8017, 11.2244)
  line L346 (-37.8017, 10.8424) -> (-37.8017, 11.6476)
  line L347 (-36.5733, 12.1137) -> (-37.3785, 12.1137)
  line L348 (-37.3785, 12.1137) -> (-37.8017, 12.5369)
  line L349 (-37.8017, 12.5369) -> (-37.3785, 12.9602)
  line L350 (-37.3785, 12.9602) -> (-36.5733, 12.9602)
  line L351 (-37.1661, 12.1137) -> (-37.1661, 12.9602)
  line L352 (-36.5733, 13.4262) -> (-37.8017, 13.4262)
  line L353 (-37.8017, 13.4262) -> (-37.8017, 14.0618)
  line L354 (-37.8017, 14.0618) -> (-37.5894, 14.2728)
  line L355 (-37.5894, 14.2728) -> (-37.1661, 14.2728)
  line L356 (-37.1661, 14.2728) -> (-36.9965, 14.0618)
  line L357 (-36.9965, 14.0618) -> (-36.9965, 13.4262)
  line L358 (-36.9965, 13.8495) -> (-36.5733, 14.2728)
  line L359 (-36.5733, 15.1621) -> (-37.8017, 15.1621)
  line L360 (-37.8017, 14.7388) -> (-37.8017, 15.544)
  line L361 (-38.4373, -2.2446) -> (-39.6658, -2.2446)
  line L362 (-39.6658, -2.2446) -> (-39.6658, -1.6517)
  line L363 (-39.6658, -1.6517) -> (-39.4535, -1.4408)
  line L364 (-39.4535, -1.4408) -> (-39.2839, -1.4408)
  line L365 (-39.2839, -1.4408) -> (-39.0729, -1.6517)
  line L366 (-39.0729, -1.6517) -> (-38.8606, -1.4408)
  line L367 (-38.8606, -1.4408) -> (-38.6483, -1.4408)
  line L368 (-38.6483, -1.4408) -> (-38.4373, -1.6517)
  line L369 (-38.4373, -1.6517) -> (-38.4373, -2.2446)
  line L370 (-39.0729, -2.2446) -> (-39.0729, -1.6517)
  line L371 (-38.4373, -0.932) -> (-39.2839, -0.932)
  line L372 (-39.2839, -0.932) -> (-39.6658, -0.5515)
  line L373 (-39.6658, -0.5515) -> (-39.2839, -0.1268)
  line L374 (-39.2839, -0.1268) -> (-38.4373, -0.1268)
  line L375 (-39.0729, -0.932) -> (-39.0729, -0.1268)
  line L376 (-38.4373, 0.7624) -> (-39.6658, 0.7624)
  line L377 (-39.6658, 0.3805) -> (-39.6658, 1.1857)
  line L378 (-38.4373, 2.075) -> (-39.6658, 2.075)
  line L379 (-39.6658, 1.6517) -> (-39.6658, 2.4983)
  line L380 (-37.5481, -2.9657) -> (-37.5481, -3.3462)
  line L381 (-37.5481, -3.3462) -> (-37.3357, -3.5585)
  line L382 (-37.3357, -3.5585) -> (-36.5305, -3.5585)
  line L383 (-36.5305, -3.5585) -> (-36.3196, -3.3462)
  line L384 (-36.3196, -3.3462) -> (-36.3196, -2.9657)
  line L385 (-36.3196, -2.9657) -> (-36.5305, -2.7534)
  line L386 (-36.5305, -2.7534) -> (-37.3357, -2.7534)
  line L387 (-37.3357, -2.7534) -> (-37.5481, -2.9657)
  line L388 (-36.3196, -2.2446) -> (-37.5481, -2.2446)
  line L389 (-37.5481, -2.2446) -> (-36.3196, -1.4408)
  line L390 (-36.3196, -1.4408) -> (-37.5481, -1.4408)
  line L391 (-36.3196, -0.932) -> (-37.5481, -0.1268)
  line L392 (-37.5481, 0.9734) -> (-37.5481, 0.5501)
  line L393 (-37.5481, 0.5501) -> (-37.3357, 0.3805)
  line L394 (-37.3357, 0.3805) -> (-36.5305, 0.3805)
  line L395 (-36.5305, 0.3805) -> (-36.3196, 0.5501)
  line L396 (-36.3196, 0.5501) -> (-36.3196, 0.9734)
  line L397 (-36.3196, 0.9734) -> (-36.5305, 1.1857)
  line L398 (-36.5305, 1.1857) -> (-37.3357, 1.1857)
  line L399 (-37.3357, 1.1857) -> (-37.5481, 0.9734)
  line L400 (-36.3196, 1.6517) -> (-37.5481, 1.6517)
  line L401 (-37.5481, 1.6517) -> (-37.5481, 2.4983)
  line L402 (-36.9124, 1.6517) -> (-36.9124, 2.075)
  line L403 (-36.3196, 2.9643) -> (-37.5481, 2.9643)
  line L404 (-37.5481, 2.9643) -> (-37.5481, 3.8122)
  line L405 (-36.9124, 2.9643) -> (-36.9124, 3.3876)
  line L406 (-36.6588, -14.6974) -> (-37.8858, -14.6974)
  line L407 (-37.8858, -14.6974) -> (-37.8858, -14.0618)
  line L408 (-37.8858, -14.0618) -> (-37.6749, -13.8922)
  line L409 (-37.6749, -13.8922) -> (-37.293, -13.8922)
  line L410 (-37.293, -13.8922) -> (-37.082, -14.0618)
  line L411 (-37.082, -14.0618) -> (-37.082, -14.6974)
  line L412 (-37.082, -14.2741) -> (-36.6588, -13.8922)
  line L413 (-37.8858, -12.5797) -> (-37.8858, -13.3849)
  line L414 (-37.8858, -13.3849) -> (-36.6588, -13.3849)
  line L415 (-36.6588, -13.3849) -> (-36.6588, -12.5797)
  line L416 (-37.293, -13.3849) -> (-37.293, -12.9616)
  line L417 (-37.6749, -11.2671) -> (-37.8858, -11.4367)
  line L418 (-37.8858, -11.4367) -> (-37.8858, -11.86)
  line L419 (-37.8858, -11.86) -> (-37.6749, -12.0709)
  line L420 (-37.6749, -12.0709) -> (-37.5053, -12.0709)
  line L421 (-37.5053, -12.0709) -> (-37.293, -11.86)
  line L422 (-37.293, -11.86) -> (-37.293, -11.4367)
  line L423 (-37.293, -11.4367) -> (-37.082, -11.2671)
  line L424 (-37.082, -11.2671) -> (-36.8697, -11.2671)
  line L425 (-36.8697, -11.2671) -> (-36.6588, -11.4367)
  line L426 (-36.6588, -11.4367) -> (-36.6588, -11.86)
  line L427 (-36.6588, -11.86) -> (-36.8697, -12.0709)
  line L428 (-37.8858, -9.9532) -> (-37.8858, -10.7583)
  line L429 (-37.8858, -10.7583) -> (-36.6588, -10.7583)
  line L430 (-36.6588, -10.7583) -> (-36.6588, -9.9532)
  line L431 (-37.293, -10.7583) -> (-37.293, -10.3351)
  line L432 (-36.6588, -9.0225) -> (-37.8858, -9.0225)
  line L433 (-37.8858, -9.4458) -> (-37.8858, -8.6406)
  line L434 (-30.4323, 55.6971) -> (-30.4323, 61.7953)
  line L435 (-30.4323, 61.7953) -> (-28.2291, 61.7953)
  line L436 (-28.2291, 61.7953) -> (-28.2291, 55.6971)
  line L437 (-28.2291, 55.6971) -> (-30.4323, 55.6971)
  line L438 (-30.22, 57.9417) -> (-28.4414, 57.9417)
  line L439 (-29.3307, 59.4666) -> (-30.22, 57.9417)
  line L440 (-28.4414, 57.9417) -> (-29.3307, 59.4666)
  line L441 (-30.22, 59.4666) -> (-29.3307, 59.4666)
  line L442 (-29.3307, 59.4666) -> (-28.4414, 59.4666)
  line L443 (-35.2607, 55.7385) -> (-35.2607, 61.8381)
  line L444 (-35.2607, 61.8381) -> (-33.0575, 61.8381)
  line L445 (-33.0575, 61.8381) -> (-33.0575, 55.7385)
  line L446 (-33.0575, 55.7385) -> (-35.2607, 55.7385)
  line L447 (-35.0484, 57.9831) -> (-33.2698, 57.9831)
  line L448 (-34.1591, 59.508) -> (-35.0484, 57.9831)
  line L449 (-33.2698, 57.9831) -> (-34.1591, 59.508)
  line L450 (-35.0484, 59.508) -> (-34.1591, 59.508)
  line L451 (-34.1591, 59.508) -> (-33.2698, 59.508)
  line L452 (-28.4414, -55.9508) -> (-28.4414, -62.0504)
  line L453 (-28.4414, -62.0504) -> (-30.6433, -62.0504)
  line L454 (-30.6433, -62.0504) -> (-30.6433, -55.9508)
  line L455 (-30.6433, -55.9508) -> (-28.4414, -55.9508)
  line L456 (-28.6524, -58.1968) -> (-30.4323, -58.1968)
  line L457 (-29.5431, -59.7203) -> (-28.6524, -58.1968)
  line L458 (-30.4323, -58.1968) -> (-29.5431, -59.7203)
  line L459 (-28.6524, -59.7203) -> (-29.5431, -59.7203)
  line L460 (-29.5431, -59.7203) -> (-30.4323, -59.7203)
  line L461 (-32.8038, -55.9095) -> (-32.8038, -62.0077)
  line L462 (-32.8038, -62.0077) -> (-35.0056, -62.0077)
  line L463 (-35.0056, -62.0077) -> (-35.0056, -55.9095)
  line L464 (-35.0056, -55.9095) -> (-32.8038, -55.9095)
  line L465 (-33.0161, -58.1541) -> (-34.7947, -58.1541)
  line L466 (-33.9054, -59.679) -> (-33.0161, -58.1541)
  line L467 (-34.7947, -58.1541) -> (-33.9054, -59.679)
  line L468 (-33.0161, -59.679) -> (-33.9054, -59.679)
  line L469 (-33.9054, -59.679) -> (-34.7947, -59.679)
  line L470 (-17.3867, 23.8454) -> (-17.3867, 17.7458)
  line L471 (-17.3867, 17.7458) -> (-19.5885, 17.7458)
  line L472 (-19.5885, 17.7458) -> (-19.5885, 23.8454)
  line L473 (-19.5885, 23.8454) -> (-17.3867, 23.8454)
  line L474 (-17.599, 21.6008) -> (-19.3776, 21.6008)
  line L475 (-18.4883, 20.0759) -> (-17.599, 21.6008)
  line L476 (-19.3776, 21.6008) -> (-18.4883, 20.0759)
  line L477 (-17.599, 20.0759) -> (-18.4883, 20.0759)
  line L478 (-18.4883, 20.0759) -> (-19.3776, 20.0759)
  line L479 (-53.303, -28.2519) -> (-62.706, -28.2519)
  line L480 (-53.303, -32.1482) -> (-53.1348, -32.1054)
  line L481 (-53.1348, -32.1054) -> (-53.0065, -31.9359)
  line L482 (-53.0065, -31.9359) -> (-52.9224, -31.7663)
  line L483 (-62.706, -28.2519) -> (-62.9183, -28.2932)
  line L484 (-62.9183, -28.2932) -> (-63.0452, -28.4201)
  line L485 (-63.0452, -28.4201) -> (-63.0879, -28.6324)
  line L486 (-52.9224, -28.6324) -> (-53.0065, -28.4201)
  line L487 (-53.0065, -28.4201) -> (-53.1348, -28.2932)
  line L488 (-53.1348, -28.2932) -> (-53.303, -28.2519)
  line L489 (-63.0879, -31.7663) -> (-63.0452, -31.9359)
  line L490 (-63.0452, -31.9359) -> (-62.9183, -32.1054)
  line L491 (-62.9183, -32.1054) -> (-62.706, -32.1482)
  line L492 (-62.706, -32.1482) -> (-53.303, -32.1482)
  line L493 (-52.9224, -31.7663) -> (-52.9224, -28.6324)
  line L494 (-63.0879, -28.6324) -> (-63.0879, -29.6913)
  line L495 (-63.0879, -29.6913) -> (-63.0879, -30.7074)
  line L496 (-63.0879, -30.7074) -> (-63.0879, -31.7663)
  line L497 (-63.0879, -30.7074) -> (-62.8756, -30.666)
  line L498 (-62.8756, -30.666) -> (-62.706, -30.4965)
  line L499 (-62.706, -30.4965) -> (-62.6219, -30.2841)
  line L500 (-62.6219, -30.2841) -> (-62.6219, -30.0718)
  line L501 (-62.6219, -30.0718) -> (-62.706, -29.8609)
  line L502 (-62.706, -29.8609) -> (-62.8756, -29.734)
  line L503 (-62.8756, -29.734) -> (-63.0879, -29.6913)
  line L504 (-63.0879, -31.809) -> (-52.9224, -31.809)
  line L505 (-71.0074, -11.9868) -> (-63.0024, -11.9868)
  line L506 (-63.0024, -11.9868) -> (-54.9974, -11.9868)
  line L507 (-54.9974, -11.9868) -> (-46.9924, -11.9868)
  line L508 (-46.9924, -11.9868) -> (-46.9924, 12.0282)
  line L509 (-46.9924, 12.0282) -> (-54.9974, 12.0282)
  line L510 (-54.9974, 12.0282) -> (-63.0024, 12.0282)
  line L511 (-63.0024, 12.0282) -> (-64.9933, 12.0282)
  line L512 (-64.9933, 12.0282) -> (-71.0074, 6.0141)
  line L513 (-71.0074, 6.0141) -> (-71.0074, -11.9868)
  line L514 (-54.9974, 12.4942) -> (-55.0829, 13.2994)
  line L515 (-55.0829, 13.2994) -> (-55.2939, 14.0191)
  line L516 (-55.2939, 14.0191) -> (-55.6758, 14.7388)
  line L517 (-55.6758, 14.7388) -> (-56.1832, 15.3316)
  line L518 (-56.1832, 15.3316) -> (-56.7774, 15.8404)
  line L519 (-56.7774, 15.8404) -> (-57.4544, 16.2209)
  line L520 (-57.4544, 16.2209) -> (-58.2168, 16.4333)
  line L521 (-58.2168, 16.4333) -> (-58.9793, 16.5187)
  line L522 (-58.9793, 16.5187) -> (-59.7844, 16.4333)
  line L523 (-59.7844, 16.4333) -> (-60.5042, 16.2209)
  line L524 (-60.5042, 16.2209) -> (-61.2239, 15.8404)
  line L525 (-61.2239, 15.8404) -> (-61.8167, 15.3316)
  line L526 (-61.8167, 15.3316) -> (-62.3255, 14.7388)
  line L527 (-62.3255, 14.7388) -> (-62.706, 14.0191)
  line L528 (-62.706, 14.0191) -> (-62.9183, 13.2994)
  line L529 (-62.9183, 13.2994) -> (-63.0024, 12.4942)
  line L530 (-63.0024, -12.4956) -> (-62.9183, -13.258)
  line L531 (-62.9183, -13.258) -> (-62.706, -14.0205)
  line L532 (-62.706, -14.0205) -> (-62.3255, -14.6974)
  line L533 (-62.3255, -14.6974) -> (-61.8167, -15.333)
  line L534 (-61.8167, -15.333) -> (-61.2239, -15.799)
  line L535 (-61.2239, -15.799) -> (-60.5042, -16.1796)
  line L536 (-60.5042, -16.1796) -> (-59.7844, -16.3919)
  line L537 (-59.7844, -16.3919) -> (-58.9793, -16.476)
  line L538 (-58.9793, -16.476) -> (-58.2168, -16.3919)
  line L539 (-58.2168, -16.3919) -> (-57.4544, -16.1796)
  line L540 (-57.4544, -16.1796) -> (-56.7774, -15.799)
  line L541 (-56.7774, -15.799) -> (-56.1832, -15.333)
  line L542 (-56.1832, -15.333) -> (-55.6758, -14.6974)
  line L543 (-55.6758, -14.6974) -> (-55.2939, -14.0205)
  line L544 (-55.2939, -14.0205) -> (-55.0829, -13.258)
  line L545 (-55.0829, -13.258) -> (-54.9974, -12.4956)
  line L546 (-63.0024, 12.4942) -> (-63.0024, 12.0282)
  line L547 (-54.9974, 12.4942) -> (-54.9974, 12.0282)
  line L548 (-63.0024, -12.4956) -> (-63.0024, -11.9868)
  line L549 (-54.9974, -12.4956) -> (-54.9974, -11.9868)
  line L550 (-48.9834, 22.9988) -> (-40.9784, 22.9988)
  line L551 (-40.9784, 22.9988) -> (-32.9734, 22.9988)
  line L552 (-32.9734, 22.9988) -> (-25.0111, 22.9988)
  line L553 (-25.0111, 22.9988) -> (-25.0111, 47.0138)
  line L554 (-25.0111, 47.0138) -> (-32.9734, 47.0138)
  line L555 (-32.9734, 47.0138) -> (-40.9784, 47.0138)
  line L556 (-40.9784, 47.0138) -> (-43.012, 47.0138)
  line L557 (-43.012, 47.0138) -> (-48.9834, 40.9997)
  line L558 (-48.9834, 40.9997) -> (-48.9834, 22.9988)
  line L559 (-32.9734, 47.5226) -> (-33.0575, 48.285)
  line L560 (-33.0575, 48.285) -> (-33.3126, 49.0461)
  line L561 (-33.3126, 49.0461) -> (-33.6503, 49.7244)
  line L562 (-33.6503, 49.7244) -> (-34.1591, 50.3173)
  line L563 (-34.1591, 50.3173) -> (-34.752, 50.826)
  line L564 (-34.752, 50.826) -> (-35.4717, 51.2066)
  line L565 (-35.4717, 51.2066) -> (-36.1927, 51.4189)
  line L566 (-36.1927, 51.4189) -> (-36.9965, 51.503)
  line L567 (-36.9965, 51.503) -> (-37.759, 51.4189)
  line L568 (-37.759, 51.4189) -> (-38.5214, 51.2066)
  line L569 (-38.5214, 51.2066) -> (-39.1998, 50.826)
  line L570 (-39.1998, 50.826) -> (-39.8354, 50.3173)
  line L571 (-39.8354, 50.3173) -> (-40.3, 49.7244)
  line L572 (-40.3, 49.7244) -> (-40.6819, 49.0461)
  line L573 (-40.6819, 49.0461) -> (-40.8943, 48.285)
  line L574 (-40.8943, 48.285) -> (-40.9784, 47.5226)
  line L575 (-40.9784, 22.4901) -> (-40.8943, 21.7276)
  line L576 (-40.8943, 21.7276) -> (-40.6819, 20.9652)
  line L577 (-40.6819, 20.9652) -> (-40.3, 20.2882)
  line L578 (-40.3, 20.2882) -> (-39.8354, 19.6954)
  line L579 (-39.8354, 19.6954) -> (-39.1998, 19.1866)
  line L580 (-39.1998, 19.1866) -> (-38.5214, 18.8047)
  line L581 (-38.5214, 18.8047) -> (-37.759, 18.5938)
  line L582 (-37.759, 18.5938) -> (-36.9965, 18.5083)
  line L583 (-36.9965, 18.5083) -> (-36.1927, 18.5938)
  line L584 (-36.1927, 18.5938) -> (-35.4717, 18.8047)
  line L585 (-35.4717, 18.8047) -> (-34.752, 19.1866)
  line L586 (-34.752, 19.1866) -> (-34.1591, 19.6954)
  line L587 (-34.1591, 19.6954) -> (-33.6503, 20.2882)
  line L588 (-33.6503, 20.2882) -> (-33.3126, 20.9652)
  line L589 (-33.3126, 20.9652) -> (-33.0575, 21.7276)
  line L590 (-33.0575, 21.7276) -> (-32.9734, 22.4901)
  line L591 (-40.9784, 47.5226) -> (-40.9784, 47.0138)
  line L592 (-32.9734, 47.5226) -> (-32.9734, 47.0138)
  line L593 (-40.9784, 22.4901) -> (-40.9784, 22.9988)
  line L594 (-32.9734, 22.4901) -> (-32.9734, 22.9988)
  line L595 (48.01, 47.0138) -> (40.005, 47.0138)
  line L596 (40.005, 47.0138) -> (32, 47.0138)
  line L597 (32, 47.0138) -> (23.995, 47.0138)
  line L598 (23.995, 47.0138) -> (23.995, 22.9988)
  line L599 (23.995, 22.9988) -> (32, 22.9988)
  line L600 (32, 22.9988) -> (40.005, 22.9988)
  line L601 (40.005, 22.9988) -> (41.9959, 22.9988)
  line L602 (41.9959, 22.9988) -> (48.01, 29.0129)
  line L603 (48.01, 29.0129) -> (48.01, 47.0138)
  line L604 (32, 22.4901) -> (32.0841, 21.7276)
  line L605 (32.0841, 21.7276) -> (32.3378, 20.9652)
  line L606 (32.3378, 20.9652) -> (32.6769, 20.2882)
  line L607 (32.6769, 20.2882) -> (33.1857, 19.6954)
  line L608 (33.1857, 19.6954) -> (33.7786, 19.1866)
  line L609 (33.7786, 19.1866) -> (34.4983, 18.8047)
  line L610 (34.4983, 18.8047) -> (35.218, 18.5938)
  line L611 (35.218, 18.5938) -> (36.0232, 18.5083)
  line L612 (36.0232, 18.5083) -> (36.7856, 18.5938)
  line L613 (36.7856, 18.5938) -> (37.548, 18.8047)
  line L614 (37.548, 18.8047) -> (38.225, 19.1866)
  line L615 (38.225, 19.1866) -> (38.8606, 19.6954)
  line L616 (38.8606, 19.6954) -> (39.3266, 20.2882)
  line L617 (39.3266, 20.2882) -> (39.7085, 20.9652)
  line L618 (39.7085, 20.9652) -> (39.9195, 21.7276)
  line L619 (39.9195, 21.7276) -> (40.005, 22.4901)
  line L620 (40.005, 47.5226) -> (39.9195, 48.285)
  line L621 (39.9195, 48.285) -> (39.7085, 49.0461)
  line L622 (39.7085, 49.0461) -> (39.3266, 49.7244)
  line L623 (39.3266, 49.7244) -> (38.8606, 50.3173)
  line L624 (38.8606, 50.3173) -> (38.225, 50.826)
  line L625 (38.225, 50.826) -> (37.548, 51.2066)
  line L626 (37.548, 51.2066) -> (36.7856, 51.4189)
  line L627 (36.7856, 51.4189) -> (36.0232, 51.503)
  line L628 (36.0232, 51.503) -> (35.218, 51.4189)
  line L629 (35.218, 51.4189) -> (34.4983, 51.2066)
  line L630 (34.4983, 51.2066) -> (33.7786, 50.826)
  line L631 (33.7786, 50.826) -> (33.1857, 50.3173)
  line L632 (33.1857, 50.3173) -> (32.6769, 49.7244)
  line L633 (32.6769, 49.7244) -> (32.3378, 49.0461)
  line L634 (32.3378, 49.0461) -> (32.0841, 48.285)
  line L635 (32.0841, 48.285) -> (32, 47.5226)
  line L636 (40.005, 22.4901) -> (40.005, 22.9988)
  line L637 (32, 22.4901) -> (32, 22.9988)
  line L638 (40.005, 47.5226) -> (40.005, 47.0138)
  line L639 (32, 47.5226) -> (32, 47.0138)
  line L640 (48.01, -22.9988) -> (40.005, -22.9988)
  line L641 (40.005, -22.9988) -> (32, -22.9988)
  line L642 (32, -22.9988) -> (23.995, -22.9988)